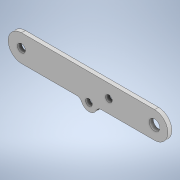
# Autodesk Inventor part: ramie_napinacza
Saved by Autodesk Inventor 2020.3 (Build 243373000, 373)
## iProperties
Created: 2021-10-24
Part Number: ramie_napinacza
Material: Ogólny
Document SubType Name: Modeling
Designer: patry
Density: 1 g/cm^3
Appearance: Domyślna
Author: patry
Autodesk Inventor part; units mm, degrees
ref_plane "YZ Plane" through (0, 0, 0) normal (1, 0, 0) x (0, 1, 0)
ref_plane "XZ Plane" through (0, 0, 0) normal (0, 1, 0) x (-1, 0, 0)
ref_plane "XY Plane" through (0, 0, 0) normal (0, 0, 1) x (1, 0, 0)
sketch "Szkic1" plane through (0, 0, 0) normal (0, 0, 1) x (1, 0, 0)
  line L0 (0, 0) -> (100, 0) construction
  line L1 (0, -10) -> (5.8348, -10)
  line L2 (100, 10) -> (0, 10)
  arc A0 (0, 10) -> (0, -10) centre (0, 0) ccw
  arc A1 (100, -10) -> (100, 10) centre (100, 0) ccw
  line L3 (5.8348, -10) -> (41.5848, -10)
  arc A2 (45.2509, -12.4) -> (56.2491, -12.4) centre (50.75, -10) ccw
  line L4 (59.9152, -10) -> (100, -10)
  arc A3 (45.2509, -12.4) -> (41.5848, -10) centre (41.5848, -14) ccw
  arc A4 (59.9152, -10) -> (56.2491, -12.4) centre (59.9152, -14) ccw
  point P0 (50, 0)
  point P1 (65.75, 0)
  point P2 (56.75, -10)
  point P3 (44.75, -10)
  dimension "d0" = 100
  dimension "d1" = 20
  dimension "d11" = 34.25
  dimension "d22" = 15
  dimension "d23" = 12
  dimension "d24" = 4
  constraints: 12 end point, 12 point on circle, 12 tangent, 5 centre point, 4 point on line, 3 coincident, 3 parallel, 1 equal radius, 1 horizontal, 1 midpoint
  measures "d0" distance of L0.start L0.end
  measures "d1" diameter of A1
  measures "d11" distance of point (100, 0) point (65.75, 0)
  measures "d22" horizontal distance of point (50.75, -10) point (65.75, 0)
  measures "d23" diameter of A2
  measures "d24" radius of A3
extrude "Wyciągnięcie proste1" add sketch "Szkic1" along normal blind 3
hole "Otwór1" at (100, 0, 0) direction (0, 0, 1) diameter 8 end through all
hole "Otwór2" at (65.75, 0, 0) at (50.75, -10, 0) direction (0, 0, 1) diameter 5 end through all
hole "Otwór3" at (0, 0, 0) direction (0, 0, 1) diameter 6 end through all
